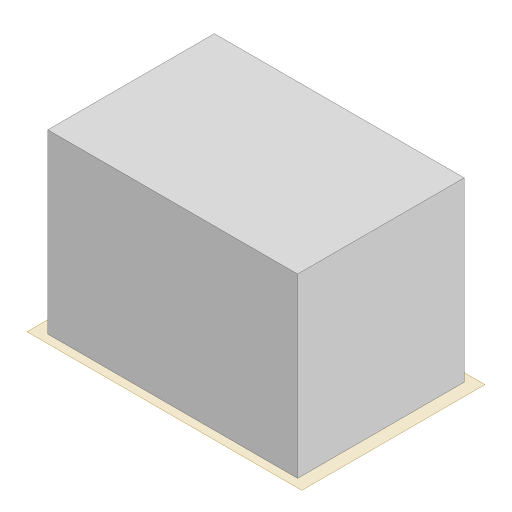
# Autodesk Inventor part: Korpus
Saved by Autodesk Inventor 2023.2 (Build 272271030, 271C)
## iProperties
Created: 2024-12-20
Part Number: Korpus
Material: Типовые
Document SubType Name: Modeling
Designer: I9232
Density: 1 g/cm^3
Appearance: По умолчанию
Author: I9232
Autodesk Inventor part; units mm, degrees
ref_plane "YZ Plane" through (0, 0, 0) normal (1, 0, 0) x (0, 1, 0)
ref_plane "XY Plane" through (0, 0, 0) normal (0, 0, 1) x (1, 0, 0)
sketch "Эскиз1" plane through (0, 0, 0) normal (0, 1, 0) x (-1, 0, 0)
  line L0 (300, 200) -> (-300, 200)
  line L1 (-300, 200) -> (-300, -200)
  line L2 (-300, -200) -> (300, -200)
  line L3 (300, -200) -> (300, 200)
  line L4 (300, 200) -> (-300, -200) construction
  line L5 (-300, 200) -> (300, -200) construction
  point P0 (0, 0)
  dimension "d0" = 600
  dimension "d1" = 400
  constraints: 12 end point, 2 midpoint, 2 parallel, 1 horizontal, 1 perpendicular
  measures "d0" distance of L1.end L2.end
  measures "d1" distance of L0.end L1.end
extrude "Выдавливание1" add sketch "Эскиз1" along normal blind 425
